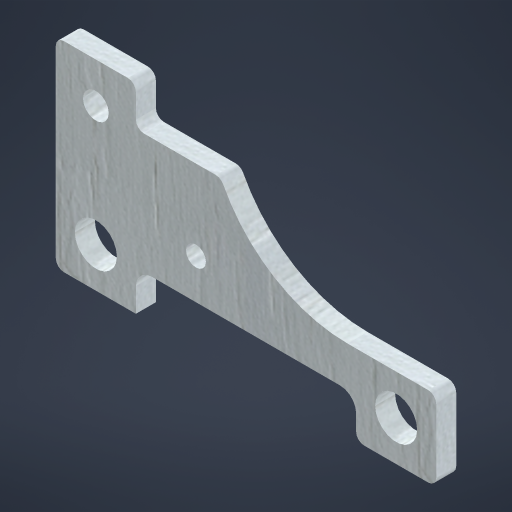
# Autodesk Inventor part: Barrel Support
Saved by Autodesk Inventor 2024.1 (Build 281209000, 209)
## iProperties
Created: 2023-10-20
Part Number: Barrel Support
Material: Wood (Walnut)
Document SubType Name: Modeling
Designer: LEGION SMIT
Density: 0.55 g/cm^3
Appearance: Wood - Painted White
Author: LEGION SMIT
Autodesk Inventor part; units mm, degrees
ref_plane "YZ Plane" through (0, 0, 0) normal (1, 0, 0) x (0, 1, 0)
ref_plane "XZ Plane" through (0, 0, 0) normal (0, 1, 0) x (-1, 0, 0)
ref_plane "XY Plane" through (0, 0, 0) normal (0, 0, 1) x (1, 0, 0)
sketch "Sketch1" plane through (0, 0, 0) normal (0, 1, 0) x (-1, 0, 0)
  line L0 (0, 2) -> (0, 48)
  line L1 (-2, 50) -> (-18, 50)
  line L2 (-20, 48) -> (-20, 42)
  line L3 (-22, 40) -> (-40, 40)
  line L4 (-2, 0) -> (-20, 0)
  line L5 (-20, 0) -> (-20, 6)
  line L6 (-24, 10) -> (-71, 10)
  line L7 (-75, 6) -> (-75, 2)
  line L8 (-77, 0) -> (-93, 0)
  line L9 (-95, 2) -> (-95, 18)
  arc A0 (-72.8634, 20) -> (-41.7764, 38.9189) centre (-72.8634, 55) ccw
  arc A1 (-40, 40) -> (-41.7764, 38.9189) centre (-40, 38) ccw
  line L10 (-93, 20) -> (-72.8634, 20)
  arc A2 (0, 48) -> (-2, 50) centre (-2, 48) ccw
  arc A3 (-2, 0) -> (0, 2) centre (-2, 2) ccw
  arc A4 (-18, 50) -> (-20, 48) centre (-18, 48) ccw
  arc A5 (-22, 40) -> (-20, 42) centre (-22, 42) ccw
  arc A6 (-77, 0) -> (-75, 2) centre (-77, 2) ccw
  arc A7 (-95, 2) -> (-93, 0) centre (-93, 2) ccw
  arc A8 (-93, 20) -> (-95, 18) centre (-93, 18) ccw
  arc A9 (-20, 6) -> (-24, 10) centre (-24, 6) ccw
  arc A10 (-71, 10) -> (-75, 6) centre (-71, 6) ccw
  circle A11 centre (-10, 40) radius 3.225
  circle A12 centre (-10, 10) radius 5.25
  circle A13 centre (-35, 20) radius 2.5
  circle A14 centre (-85, 10) radius 5.25
  point P0 (0, 0)
  point P1 (0, 50)
  point P2 (-20, 50)
  point P3 (-20, 40)
  point P4 (-20, 10)
  point P5 (-75, 10)
  point P6 (-75, 0)
  point P7 (-95, 0)
  point P8 (-95, 20)
  dimension "d0" = 50
  dimension "d1" = 20
  dimension "d2" = 10
  dimension "d3" = 20
  dimension "d4" = 20
  dimension "d5" = 10
  dimension "d6" = 55
  dimension "d7" = 20
  dimension "d8" = 20
  dimension "d9" = 70
  dimension "d11" = 4
  dimension "d12" = 2
  dimension "d13" = 2
  dimension "d14" = 4
  dimension "d15" = 6.45
  dimension "d16" = 10.5
  dimension "d17" = 30
  dimension "d18" = 10
  dimension "d19" = 10
  dimension "d20" = 10
  dimension "d21" = 5
  dimension "d22" = 25
  dimension "d25" = 10.5
  dimension "d26" = 10
  constraints: 22 end point, 22 point on circle, 21 point on line, 20 tangent, 15 centre point, 7 perpendicular, 6 equal radius, 2 horizontal, 1 horizontal alignment, 1 vertical, 1 vertical alignment
  measures "d0" distance of point (0, 0) point (0, 50)
  measures "d1" distance of point (0, 50) point (-20, 50)
  measures "d2" distance of point (-20, 50) point (-20, 40)
  measures "d3" distance of point (-20, 40) L3.end
  measures "d4" distance of point (0, 0) L4.end
  measures "d5" distance of L4.end point (-20, 10)
  measures "d6" distance of point (-20, 10) point (-75, 10)
  measures "d7" distance of point (-75, 0) point (-95, 0)
  measures "d8" distance of point (-95, 0) point (-95, 20)
  measures "d9" diameter of A0
  measures "d11" diameter of A1
  measures "d12" radius of A2
  measures "d13" radius of A6
  measures "d14" radius of A9
  measures "d15" diameter of A11
  measures "d16" diameter of A12
  measures "d17" distance of A12.centre A11.centre
  measures "d18" distance from line of A11.centre L0
  measures "d19" distance from line of L4 A12.centre
  measures "d20" distance from line of A12.centre L5
  measures "d21" diameter of A13
  measures "d22" horizontal distance of A13.centre A11.centre
  measures "d25" diameter of A14
  measures "d26" distance from line of A14.centre L9
extrude "Extrusion1" add sketch "Sketch1" along normal blind 5
body "Solid1"
